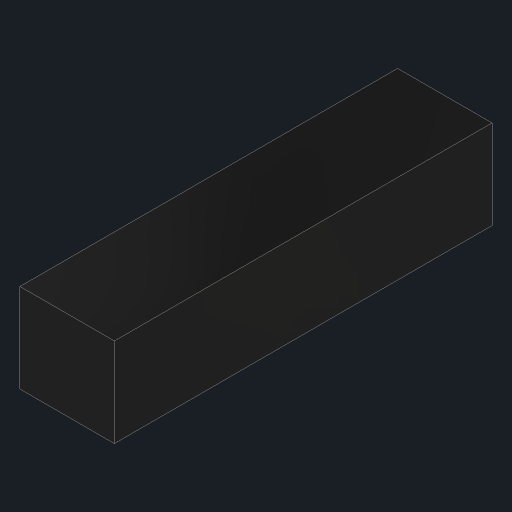
# Autodesk Inventor part: smolLipo
Saved by Autodesk Inventor 2023 (Build 270158000, 158)
## iProperties
Created: 2024-04-13
Part Number: smolLipo
Material: Acetal Resin, Black
Document SubType Name: Modeling
Designer: szymo
Density: 1.425 g/cm^3
Appearance: Smooth - Black
Mass: 35 g
Surface Area: 46.96 cm^2
Volume: 16.32 cm^3
Author: szymo
Autodesk Inventor part; units mm, degrees
ref_plane "YZ Plane" through (0, 0, 0) normal (1, 0, 0) x (0, 1, 0)
ref_plane "XZ Plane" through (0, 0, 0) normal (0, 1, 0) x (-1, 0, 0)
ref_plane "XY Plane" through (0, 0, 0) normal (0, 0, 1) x (1, 0, 0)
sketch "Sketch1" plane through (0, 0, 0) normal (0, 1, 0) x (-1, 0, 0)
  line L0 (0, 0) -> (-15, 0)
  line L1 (-15, 0) -> (-15, -68)
  line L2 (-15, -68) -> (0, -68)
  line L3 (0, -68) -> (0, 0)
  dimension "d0" = 15
  dimension "d1" = 68
  constraints: 8 end point, 2 parallel, 1 horizontal, 1 perpendicular
  measures "d0" distance of L2.end L1.end
  measures "d1" distance of L1.end L0.end
extrude "Extrusion1" add sketch "Sketch1" along normal blind 16
sketch "Sketch3" plane through (0, 16, 0) normal (0, 1, 0) x (1, 0, 0)
  line L0 (15, 0) -> (15, 68) projected
  line L1 (15, 68) -> (0, 68) projected
  line L2 (0, 68) -> (0, 0) projected
  line L3 (0, 0) -> (15, 0) projected
  line L4 (16, 0) -> (-1, 0)
  line L5 (-1, 0) -> (-1, 68)
  line L6 (-1, 68) -> (16, 68)
  line L7 (16, 68) -> (16, 0)
  point P0 (7.5, 68)
  dimension "d6" = 0
  dimension "d7" = 0
  dimension "d8" = 1
  dimension "d9" = 1
  constraints: 8 end point, 2 parallel, 1 horizontal, 1 midpoint, 1 perpendicular
  measures "d6" distance from line of point (7.5, 68) L6
  measures "d7" distance between parallel lines of L4 L3
  measures "d8" distance between parallel lines of L2 L5
  measures "d9" distance between parallel lines of L7 L0
extrude "offset" add sketch "Sketch3" against normal up to surface (16 mm away) contours L0 L6 L7 L4 | L4 L5 L6 L2
body "Solid1"
